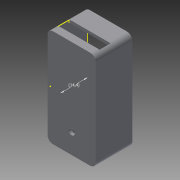
# Autodesk Inventor part: bottom v3
Saved by Autodesk Inventor 2014 (Build 180170000, 170)
## iProperties
Created: 2018-03-27
Part Number: bottom v3
Material: Generic
Document SubType Name: Modeling
Designer: HP820
Density: 1 g/cm^3
Appearance: Default
Author: HP820
Autodesk Inventor part; units mm, degrees
ref_plane "YZ Plane" through (0, 0, 0) normal (1, 0, 0) x (0, 1, 0)
ref_plane "XZ Plane" through (0, 0, 0) normal (0, 1, 0) x (-1, 0, 0)
ref_plane "XY Plane" through (0, 0, 0) normal (0, 0, 1) x (1, 0, 0)
sketch "Sketch1" plane through (0, 0, 0) normal (0, 1, 0) x (-1, 0, 0)
  line L0 (-11.5, 25) -> (11.5, 25)
  line L1 (11.5, 25) -> (11.5, -25)
  line L2 (11.5, -25) -> (-11.5, -25)
  line L3 (-11.5, -25) -> (-11.5, 25)
  line L4 (-11.5, 25) -> (11.5, -25) construction
  line L5 (11.5, 25) -> (-11.5, -25) construction
  line L6 (-13.1, -26.6) -> (13.1, -26.6)
  line L7 (13.1, -26.6) -> (13.1, 26.6)
  line L8 (13.1, 26.6) -> (-13.1, 26.6)
  line L9 (-13.1, 26.6) -> (-13.1, -26.6)
  line L10 (-13.1, -26.6) -> (13.1, 26.6) construction
  line L11 (13.1, -26.6) -> (-13.1, 26.6) construction
  point P0 (0, 0)
  dimension "d0" = 23
  dimension "d1" = 50
  dimension "d2" = 1.6
  dimension "d3" = 1.6
  constraints: 24 end point, 4 midpoint, 4 parallel, 2 horizontal, 2 perpendicular
  measures "d0" distance of L1.end L2.end
  measures "d1" distance of L0.end L1.end
  measures "d2" distance between parallel lines of L0 L8
  measures "d3" distance between parallel lines of L7 L1
extrude "Extrusion1" add sketch "Sketch1" along normal blind 20
sketch "Sketch2" plane through (0, 0, 0) normal (0, -1, 0) x (1, 0, 0)
  line L0 (-11.5, -25) -> (-11.5, 25) projected
  line L1 (-11.5, 25) -> (11.5, 25) projected
  line L2 (11.5, 25) -> (11.5, -25) projected
  line L3 (11.5, -25) -> (-11.5, -25) projected
  point P0 (0, 0)
extrude "Extrusion2" add sketch "Sketch2" against normal blind 1.6
sketch "Sketch3" plane through (0, 1.6, 0) normal (0, 1, 0) x (1, 0, 0)
  line L0 (-11.5, 25) -> (11.5, 25) projected
  line L1 (-10.5, 9) -> (10.5, 9)
  line L2 (10.5, 9) -> (10.5, -23)
  line L3 (10.5, -23) -> (-10.5, -23)
  line L4 (-10.5, -23) -> (-10.5, 9)
  line L5 (-10.5, 9) -> (10.5, -23) construction
  line L6 (10.5, 9) -> (-10.5, -23) construction
  circle A0 centre (-7, 5.5) radius 1.3
  circle A1 centre (-7, 5.5) radius 3.5
  point P0 (0, 0)
  point P1 (0, -7)
  dimension "d8" = 21
  dimension "d9" = 32
  dimension "d10" = 16
  dimension "d11" = 2.6
  dimension "d26" = 3.5
  dimension "d27" = 3.5
  dimension "d29" = 7
  constraints: 12 end point, 2 centre point, 2 midpoint, 2 parallel, 1 coincident, 1 horizontal
  measures "d8" distance of L2.end L3.end
  measures "d9" distance of L1.end L2.end
  measures "d10" distance between parallel lines of L0 L1
  measures "d11" diameter of A0
  measures "d26" distance from line of L4 A0.centre
  measures "d27" distance from line of L1 A0.centre
  measures "d29" diameter of A1
extrude "Extrusion3" add sketch "Sketch3" along normal blind 4 contours A1
sketch "Sketch4" plane through (-13.1, 0, 26.6) normal (0, 0, 1) x (1, 0, 0)
  line L0 (0, 0) -> (26.2, 0) projected
  line L1 (1.6, 1.6) -> (1.6, 20) projected
  line L2 (1.6, 1.6) -> (1.6, 20) projected
  line L3 (24.6, 1.6) -> (24.6, 20) projected
  line L4 (24.6, 1.6) -> (24.6, 20) projected
  line L5 (1.6, 4) -> (24.1799, 4)
  line L6 (24.1799, 4) -> (24.1799, 10)
  line L7 (24.1799, 10) -> (1.6, 10)
  line L8 (1.6, 10) -> (1.6, 4)
  point P0 (13.1, 0)
  dimension "d16" = 6
  dimension "d17" = 4
  constraints: 8 end point, 2 parallel, 1 horizontal, 1 perpendicular, 1 point on line
  measures "d16" distance of L6.end L5.end
  measures "d17" distance between parallel lines of L0 L5
extrude "Extrusion4" cut sketch "Sketch4" against normal blind 4
sketch "Sketch5" plane through (0, 1.6, 0) normal (0, 1, 0) x (1, 0, 0)
  line L0 (-11.5, -25) -> (-11.5, 25) projected
  line L1 (11.5, -25) -> (-11.5, -25) projected
  line L2 (11.5, 25) -> (11.5, -25) projected
  line L3 (6.8, 0) -> (8, 0)
  line L4 (8, 0) -> (8, -25)
  line L5 (8, -25) -> (6.8, -25)
  line L6 (6.8, -25) -> (6.8, 0)
  line L7 (-8, 0) -> (-6.8, 0)
  line L8 (-6.8, 0) -> (-6.8, -25)
  line L9 (-6.8, -25) -> (-8, -25)
  line L10 (-8, -25) -> (-8, 0)
  point P0 (0, 0)
  dimension "d20" = 1.2
  dimension "d21" = 1.2
  dimension "d22" = 3.5
  dimension "d23" = 3.5
  constraints: 16 end point, 4 parallel, 2 horizontal, 2 perpendicular, 2 point on line
  measures "d20" distance of L4.end L5.end
  measures "d21" distance of L8.end L9.end
  measures "d22" distance between parallel lines of L10 L0
  measures "d23" distance between parallel lines of L2 L4
extrude "Extrusion5" add sketch "Sketch5" along normal blind 4
fillet "Fillet1" radius 3 4 edges at (13.1, 10, 26.6) (13.1, 10, -26.6) (-13.1, 10, -26.6) (-13.1, 10, 26.6)
sketch "Sketch6" plane through (10.1, 0, -26.6) normal (0, 0, -1) x (-1, 0, 0)
  circle A0 centre (10.1, 10) radius 2.6
  point P0 (10.1, 0)
  dimension "d31" = 5.2
  constraints: 1 centre point
  measures "d31" diameter of A0
extrude "Extrusion6" cut sketch "Sketch6" against normal blind 4
sketch "Sketch7" plane through (10.1, 0, -26.6) normal (0, 0, -1) x (-1, 0, 0)
  circle A0 centre (10.1, 10) radius 2.6 projected
  circle A1 centre (10.1, 10) radius 4
  point P0 (10.1, 0)
  dimension "d34" = 8
  constraints: 1 centre point, 1 coincident
  measures "d34" diameter of A1
extrude "Extrusion7" add sketch "Sketch7" along normal blind 2
fillet "Fillet2" radius 3 2 edges at (4, 10, -26.6) (4, 10, -28.6)
sketch "Sketch8" plane through (-11.5, 20, 25) normal (1, 0, 0) x (0, 0, -1)
  line L0 (-1.2533, -16) -> (-1.2533, -10) projected
  line L1 (-1.2533, -16) -> (0, -16) projected
  line L2 (0, -18.4) -> (0, -16) projected
  line L3 (0, -18.4) -> (50, -18.4) projected
  line L4 (50, -18.4) -> (50, 0) projected
  line L5 (0, 0) -> (50, 0) projected
  line L6 (0, -10) -> (0, 0) projected
  line L7 (-1.2533, -10) -> (0, -10) projected
  line L8 (27, -18.4) -> (34, -18.4) projected
  line L9 (29.2, -14.4) -> (31.8, -14.4) projected
  line L10 (34, -14.4) -> (27, -14.4) projected
  point P0 (25, -20)
  dimension "d38" = 14.4
  measures "d38" distance between parallel lines of L5 L10
sketch "Sketch9" plane through (11.5, 20, 25) normal (0, 0, -1) x (-1, 0, 0)
  line L0 (23, -10) -> (23, 0) projected
  line L1 (0, 0) -> (23, 0)
  line L2 (23, 0) -> (23, -1.4)
  line L3 (23, -1.4) -> (0, -1.4)
  line L4 (0, -1.4) -> (0, 0)
  point P0 (11.5, -20)
  dimension "d39" = 1.4
  constraints: 8 end point, 2 parallel, 1 horizontal, 1 perpendicular, 1 point on line
  measures "d39" distance of L1.end L2.end
extrude "Extrusion8" add sketch "Sketch9" along normal blind 2
sketch "Sketch10" plane through (0, 1.6, 0) normal (0, 1, 0) x (1, 0, 0)
  line L0 (11.5, 25) -> (11.5, -25) projected
  line L1 (-11.5, 25) -> (11.5, 25) projected
  line L2 (-11.5, -25) -> (-11.5, 25) projected
  circle A0 centre (-8.3566, 21.8566) radius 1.2
  circle A1 centre (-8.3566, 21.8566) radius 3.1434
  circle A2 centre (8.3566, 21.8566) radius 1.2
  circle A3 centre (8.3566, 21.8566) radius 3.1434
  point P0 (0, 0)
  dimension "d45" = 2.4
  dimension "d46" = 3.1434
  dimension "d47" = 3.1434
  dimension "d48" = 2.4
  dimension "d49" = 3.1434
  dimension "d50" = 3.1434
  constraints: 4 centre point, 2 coincident, 1 tangent
  measures "d45" diameter of A0
  measures "d46" distance from line of L2 A1.centre
  measures "d47" distance from line of L1 A0.centre
  measures "d48" diameter of A2
  measures "d49" distance from line of L1 A3.centre
  measures "d50" distance from line of L0 A3.centre
extrude "Extrusion9" add sketch "Sketch10" along normal up to surface (18.4 mm away) contours A3 | A1
chamfer "Chamfer2" distance 1 angle 45 1 edges at (0, 18.6, 23)
sketch "Sketch11" plane through (0, 1.6, 0) normal (0, 1, 0) x (1, 0, 0)
  circle A0 centre (0, 15.6096) radius 1.7
  point P0 (0, 0)
  dimension "d56" = 3.4
  constraints: 1 centre point
  measures "d56" diameter of A0
extrude "Extrusion10" cut sketch "Sketch11" against normal through all
equation "\"d3\" = d2"
equation "\"d47\" = d46"
equation "\"d49\" = d47"
equation "\"d50\" = d46"
body "Solid1"
